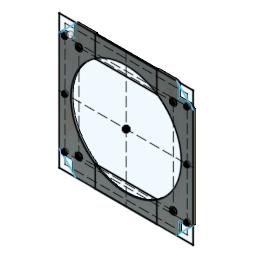
MEYTONFRAME178v17 (Autodesk Fusion 360 design; units mm, degrees)
Autodesk Fusion 360 part; units mm, degrees
sketch "Sketch1" plane through (0, 0, 0) normal (0, 1, 0) x (1, 0, 0) in component "Raam_v3"
  line L0 (-100, 100) -> (100, 100)
  line L1 (100, 100) -> (100, -100)
  line L2 (100, -100) -> (-100, -100)
  line L3 (-100, -100) -> (-100, 100)
  circle A0 centre (0, 0) radius 82.5
  line L4 (-70.5, -70.5) -> (70.5, -70.5) construction
  line L5 (70.5, -70.5) -> (70.5, 70.5) construction
  line L6 (70.5, 70.5) -> (-70.5, 70.5) construction
  line L7 (-70.5, 70.5) -> (-70.5, -70.5) construction
  line L8 (-46, -100) -> (46, -100)
  line L9 (46, -100) -> (46, -68)
  line L10 (46, -68) -> (-46, -68)
  line L11 (-46, -68) -> (-46, -100)
  line L12 (-46, 100) -> (46, 100)
  line L13 (46, 100) -> (46, 68)
  line L14 (46, 68) -> (-46, 68)
  line L15 (-46, 68) -> (-46, 100)
  circle A1 centre (70.5, -70.5) radius 5
  circle A2 centre (-70.5, -70.5) radius 5
  circle A3 centre (70.5, 70.5) radius 5
  circle A4 centre (-70.5, 70.5) radius 5
  line L16 (-91.25, -91.25) -> (91.25, -91.25) construction
  line L17 (91.25, -91.25) -> (91.25, 91.25) construction
  line L18 (91.25, 91.25) -> (-91.25, 91.25) construction
  line L19 (-91.25, 91.25) -> (-91.25, -91.25) construction
  line L20 (0, -100) -> (0, 100) construction
  line L21 (-100, 0) -> (100, 0) construction
  line L22 (-100, -75) -> (-74.4285, -100)
  line L23 (100, -75) -> (75.5588, -100)
  line L24 (-100, 75) -> (-75.5588, 100)
  line L25 (74.4285, 100) -> (100, 75)
  circle A5 centre (-91.25, 0) radius 1.5
  circle A6 centre (91.25, 0) radius 1.5
  line L26 (-100, -75) -> (100, -75) construction
  circle A7 centre (91.25, -75) radius 1.5
  line L27 (-100, 75) -> (100, 75) construction
  circle A8 centre (91.25, 75) radius 1.5
  circle A9 centre (-91.25, 75) radius 1.5
  circle A10 centre (-91.25, -75) radius 1.5
  line L28 (-95.1383, -79.753) -> (-77.6201, -79.753)
  line L29 (-77.6201, -79.753) -> (-77.6201, -96.8797)
  line L30 (-83.7274, -79.753) -> (-83.7274, -80)
  line L31 (95.3116, -79.7956) -> (78.4368, -79.7956)
  line L32 (78.4368, -79.7956) -> (78.4368, -97.0562)
  line L33 (-95.1178, 79.9938) -> (-80.1166, 79.9938)
  line L34 (-80.1166, 79.9938) -> (-80.1166, 95.3379)
  line L35 (94.9708, 79.9168) -> (79.5428, 79.9168)
  line L36 (79.5428, 79.9168) -> (79.5428, 95)
  dimension "d1" = 200
  dimension "d2" = 200
  dimension "d3" = 165
  dimension "d6" = 141
  dimension "d7" = 141
  dimension "d8" = 29.5
  dimension "d9" = 29.5
  dimension "d11" = 100
  dimension "d12" = 100
  dimension "d18" = 92
  dimension "d19" = 32
  dimension "d20" = 46
  dimension "d21" = 92
  dimension "d22" = 32
  dimension "d23" = 46
  dimension "d24" = 10
  dimension "d25" = 10
  dimension "d26" = 10
  dimension "d27" = 10
  dimension "d28" = 182.5
  dimension "d29" = 182.5
  dimension "d30" = 70.5
  dimension "d31" = 8.75
  dimension "d32" = 8.75
  dimension "d33" = 3
  dimension "d34" = 3
  dimension "d53" = 12.3744
  dimension "d54" = 12.3744
  dimension "d55" = 12.3744
  dimension "d56" = 12.3744
  dimension "d57" = 41.7193
  dimension "d58" = 41.7193
  dimension "d59" = 75
  dimension "d60" = 3
  dimension "d61" = 75
  dimension "d62" = 3
  dimension "d63" = 3
  dimension "d64" = 3
  constraint horizontal L0
  constraint vertical L1
  constraint horizontal L2
  constraint vertical L3
  constraint coincident A0.centre origin
  constraint horizontal L4
  constraint vertical L5
  constraint horizontal L6
  constraint vertical L7
  constraint horizontal L8
  constraint vertical L9
  constraint horizontal L10
  constraint vertical L11
  constraint coincident L2 L8.start
  constraint horizontal L12
  constraint vertical L13
  constraint horizontal L14
  constraint vertical L15
  constraint coincident L0 L12.start
  constraint coincident L4.end L5.start
  constraint coincident L4.start L7.end
  constraint coincident L5.end L6.start
  constraint coincident L6.end L7.start
  constraint horizontal L16
  constraint vertical L17
  constraint horizontal L18
  constraint vertical L19
  constraint midpoint L8 L20.start
  constraint midpoint L0 L20.end
  constraint midpoint L3 L21.start
  constraint midpoint L1 L21.end
  constraint coincident L3 L22.start
  constraint coincident L2 L22.end
  constraint coincident L1 L23.start
  constraint coincident L2 L23.end
  constraint perpendicular L22 L23
  constraint coincident L3 L24.start
  constraint coincident L0 L24.end
  constraint parallel L23 L24
  constraint coincident L0 L25.start
  constraint coincident L1 L25.end
  constraint perpendicular L24 L25
  constraint midpoint L19 A5.centre
  constraint midpoint L17 A6.centre
  constraint perpendicular L1 L26
  constraint coincident L17 A7.centre
  constraint coincident L26 A7.centre
  constraint perpendicular L3 L27
  constraint coincident L17 A8.centre
  constraint coincident L27 A8.centre
  constraint coincident L27 A9.centre
  constraint coincident L19 A9.centre
  constraint coincident L19 A10.centre
  constraint coincident L26 A10.centre
  constraint coincident L22 L28.start
  constraint perpendicular L19 L28
  constraint coincident L22 L29.end
  constraint perpendicular L16 L29
  constraint coincident L28 L30.start
  constraint perpendicular L28 L30
  constraint coincident L23 L31.start
  constraint perpendicular L1 L31
  constraint coincident L23 L32.end
  constraint perpendicular L16 L32
  constraint coincident L24 L33.start
  constraint perpendicular L19 L33
  constraint coincident L24 L34.end
  constraint perpendicular L18 L34
  constraint coincident L25 L35.start
  constraint parallel L18 L35
  constraint coincident L25 L36.end
  constraint perpendicular L18 L36
  measures "d1" distance of L0.start L0.end
  measures "d2" distance of L0.start L2.end
  measures "d3" diameter of A0
  measures "d6" distance of L4.start L4.end
  measures "d7" distance of L4.start L6.end
  measures "d8" horizontal distance of L1.end L4.end
  measures "d9" vertical distance of L1.end L4.end
  measures "d11" vertical distance of A0.centre L1.end
  measures "d12" horizontal distance of L2.end A0.centre
  measures "d18" distance of L8.start L8.end
  measures "d19" distance of L8.start L10.end
  measures "d20" horizontal distance of A0.centre L8.start
  measures "d21" distance of L12.start L12.end
  measures "d22" distance of L12.start L14.end
  measures "d23" horizontal distance of A0.centre L14.end
  measures "d24" diameter of A1
  measures "d25" diameter of A2
  measures "d26" diameter of A3
  measures "d27" diameter of A4
  measures "d28" distance of L16.start L16.end
  measures "d29" distance of L16.start L18.end
  measures "d30" horizontal distance of A0.centre L4.start
  measures "d31" vertical distance of L0.end L17.end
  measures "d32" horizontal distance of L0.end L17.end
  measures "d33" diameter of A5
  measures "d34" diameter of A6
  measures "d53" distance of L1.end L16.end
  measures "d54" distance of L2.end L16.start
  measures "d55" distance of L0.end L17.end
  measures "d56" distance of L0.start L18.end
  measures "d57" distance of L2.end L4.start
  measures "d58" distance of L0.end L5.end
  measures "d59" distance of L21.end L23.start
  measures "d60" diameter of A7
  measures "d61" distance of L21.end L25.end
  measures "d62" diameter of A8
  measures "d63" diameter of A9
  measures "d64" diameter of A10
extrude "Extrude11" add sketch "Sketch1" along normal blind 1.25 contours L0 A0 L12 L13 L15 | L2 A0 L8 L9 L11 makes body 1 at (0, 0, -94.1667) makes body 2 at (0, 0, 94.1667) in component "Raam_v3"
extrude "Extrude10" add sketch "Sketch1" along normal blind 2 separate body contours L0 L2 L3 A0 L11 L15 L22 L24 L28 L29 L33 L34 | L0 L1 L2 A0 L9 L13 L23 L25 L31 L32 L35 L36 makes body 3 at (-63.4107, 0, -91.7181) makes body 4 at (63.4107, 2, 91.7181) in component "Raam_v3"
extrude "Extrude12" add sketch "Sketch1" along normal blind 3.5 contours A2 bodies 3 in component "Raam_v3"
extrude "Extrude13" add sketch "Sketch1" along normal blind 3.5 contours A1 bodies 4 in component "Raam_v3"
extrude "Extrude14" add sketch "Sketch1" along normal blind 3.5 contours A4 bodies 3 in component "Raam_v3"
extrude "Extrude15" add sketch "Sketch1" along normal blind 3.5 contours A3 bodies 4 in component "Raam_v3"
extrude "Extrude16" add 1 faces at (63.4107, 2, 91.7181) along direction (0, 1, 0) blind 2 on bodies 4 bodies 4 in component "Raam_v3"
extrude "Extrude17" add 1 faces at (-63.4107, 2, -91.7181) along direction (0, 1, 0) blind 2 on bodies 3 bodies 3 in component "Raam_v3"
extrude "Extrude18" add 1 faces at (0, 1.25, 94.1667) along direction (0, 1, 0) blind 1 on bodies 2 bodies 2 3 4 in component "Raam_v3"
extrude "Extrude19" add 1 faces at (0, 1.25, -94.1667) along direction (0, 1, 0) blind 1 on bodies 1 bodies 1 2 in component "Raam_v3"
extrude "Extrude20" add 1 faces at (-69.0538, 3.5, 70.0197) along direction (0, 1, 0) blind 4 on bodies 1 bodies 1 in component "Raam_v3"
extrude "Extrude21" cut 1 faces at (-69.0538, 7.5, 70.0197) along direction (0, -1, 0) blind 1 on bodies 1 bodies 1 in component "Raam_v3"
extrude "Extrude22" add 1 faces at (71.8216, 3.5, 69.804) along direction (0, 1, 0) blind 3 on bodies 1 bodies 1 in component "Raam_v3"
extrude "Extrude23" add 1 faces at (-69.0538, 3.5, -70.9803) along direction (0, 1, 0) blind 3 on bodies 1 bodies 1 in component "Raam_v3"
extrude "Extrude24" cut 1 faces at (-63.4107, 4, -91.7181) along direction (0, -1, 0) blind 1 on bodies 1 bodies 1 in component "Raam_v3"
extrude "Extrude25" cut 1 faces at (63.4107, 4, 91.7181) along direction (0, -1, 0) blind 1 on bodies 1 bodies 1 in component "Raam_v3"
extrude "Extrude26" cut 1 faces at (0, 2.25, 94.1667) along direction (0, -1, 0) blind 0.5 on bodies 1 bodies 1 in component "Raam_v3"
extrude "Extrude27" cut 1 faces at (0, 2.25, -94.1667) along direction (0, -1, 0) blind 0.5 on bodies 1 bodies 1 in component "Raam_v3"
extrude "Extrude28" cut 1 faces at (-69.0538, 6.5, 70.0197) along direction (0, -1, 0) blind 1 on bodies 1 bodies 1 in component "Raam_v3"
extrude "Extrude29" cut 1 faces at (71.8216, 6.5, 69.804) along direction (0, -1, 0) blind 1 on bodies 1 bodies 1 in component "Raam_v3"
extrude "Extrude30" cut 1 faces at (71.8216, 3.5, -71.196) along direction (0, -1, 0) blind 1 on bodies 1 bodies 1 in component "Raam_v3"
extrude "Extrude31" cut 1 faces at (-69.0538, 6.5, -70.9803) along direction (0, -1, 0) blind 1 on bodies 1 bodies 1 in component "Raam_v3"
extrude "Extrude32" add 1 faces at (71.8216, 2.5, -71.196) along direction (0, 1, 0) blind 3 on bodies 1 bodies 1 in component "Raam_v3"
extrude "Extrude2" [suppressed] in component "Raam_v3"
extrude "Extrude1" [suppressed] in component "Raam_v3"
extrude "Extrude3" [suppressed] in component "Raam_v3"
extrude "Extrude4" [suppressed] in component "Raam_v3"
extrude "Extrude5" [suppressed] in component "Raam_v3"
extrude "Extrude6" [suppressed] in component "Raam_v3"
extrude "Extrude7" [suppressed] in component "Raam_v3"
extrude "Extrude8" [suppressed] in component "Raam_v3"
extrude "Extrude9" [suppressed] in component "Raam_v3"
hole "Hole1" [suppressed] in component "Raam_v3"
hole "Hole2" [suppressed] in component "Raam_v3"
hole "Hole3" [suppressed] in component "Raam_v3"
move_body "Move1" [suppressed] in component "Raam_v3"
move_body "Move2" [suppressed] in component "Raam_v3"
hole "Hole4" [suppressed] in component "Raam_v3"
delete_face "DeleteFace1" [suppressed] in component "Raam_v3"
delete_face "DeleteFace2" [suppressed] in component "Raam_v3"
hole "Hole5" [suppressed] in component "Raam_v3"
delete_face "DeleteFace3" [suppressed] in component "Raam_v3"
hole "Hole6" [suppressed] in component "Raam_v3"
hole "Hole7" [suppressed] in component "Raam_v3"
component "Raam_v3" placed x (1, 0, 0) y (0, 1, 0) z (0, 0, 1) at (0, 0, 0)
